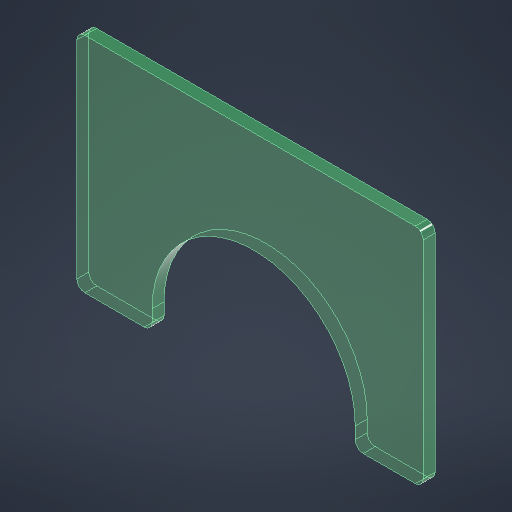
# Autodesk Inventor part: PAREDES LATERALES
Saved by Autodesk Inventor 2026.2 (Build 302298000, 298)
## iProperties
Created: 2026-02-05
Part Number: PAREDES LATERALES
Material: Generic
Document SubType Name: Modeling
Designer: 06aar
Density: 1 g/cm^3
Appearance: Clear - Green 1
Author: 06aar
Autodesk Inventor part; units mm, degrees
ref_plane "YZ Plane" through (0, 0, 0) normal (1, 0, 0) x (0, 1, 0)
ref_plane "XZ Plane" through (0, 0, 0) normal (0, 1, 0) x (-1, 0, 0)
ref_plane "XY Plane" through (0, 0, 0) normal (0, 0, 1) x (1, 0, 0)
sketch "Sketch1" plane through (0, 0, 0) normal (0, 0, 1) x (1, 0, 0)
  line L0 (2, 0) -> (20.9174, 0)
  line L1 (87, 2) -> (87, 54)
  line L2 (85, 56) -> (2, 56)
  line L3 (0, 54) -> (0, 2)
  line L4 (44.4174, 5) -> (44.4174, 0)
  arc A0 (2, 56) -> (0, 54) centre (2, 54) ccw
  arc A1 (87, 54) -> (85, 56) centre (85, 54) ccw
  arc A2 (85, 0) -> (87, 2) centre (85, 2) ccw
  arc A3 (0, 2) -> (2, 0) centre (2, 2) ccw
  line L5 (69.9174, 0) -> (85, 0)
  line L6 (20.9174, 0) -> (20.9174, 5)
  circle A4 centre (44.4174, 5) radius 23.5
  line L7 (67.9174, 0) -> (67.9174, 5)
  line L8 (67.9174, 0) -> (69.9174, 0)
  circle A5 centre (44.4174, 5) radius 25.5
  line L9 (18.9174, 5) -> (18.9174, 0)
  line L10 (69.9174, 5) -> (69.9174, 0)
  point P0 (0, 0)
  point P1 (87, 56)
  point P2 (87, 0)
  point P3 (0, 56)
  dimension "d0" = 87
  dimension "d1" = 56
  dimension "d2" = 5
  dimension "d7" = 2
  dimension "d10" = 20.9174
  dimension "d11" = 47
  dimension "d12" = 2
  constraints: 22 end point, 13 point on line, 13 tangent, 12 point on circle, 6 centre point, 4 parallel, 4 perpendicular, 3 equal radius, 2 coincident, 2 horizontal
  measures "d0" distance between parallel lines of L1 L3
  measures "d1" distance between parallel lines of L0 L2
  measures "d2" distance of L4.start L4.end
  measures "d7" radius of A0
  measures "d10" distance between parallel lines of L3 L6
  measures "d11" diameter of A4
  measures "d12" radial gap between concentric circles of A4 A5
extrude "Extrusion1" add sketch "Sketch1" along normal blind 3 contours A3 L3 A0 L2 A1 L1 A2 L5 L10 A5 L9 L0
fillet "Fillet1" radius 2 2 edges at (18.9174, 0, 1.5) (69.9174, 0, 1.5)
body "Solid1"
